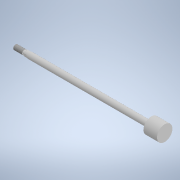
# Autodesk Inventor part: 32121200-s3
Saved by Autodesk Inventor 2024.3 (Build 283343000, 343)
## iProperties
Category: PARTsolutions
Company: METALWORK
Created: 2025-06-08
Part Number: 32121200-s3
Material: Generic
Catalog Web Link: www.cadenas.de
Description: ISO 15552 Type A rod-
Vendor: METALWORK
Document SubType Name: Modeling
Designer: psAdmin
Manufacturer: METALWORK
Mass: 53.2784 g
Surface Area: 148.649 cm^2
Volume: 53.2784 cm^3
Density: 1 g/cm^3
Appearance: PSOLRGB-175-175-175
PSOL_IDENT_0: {$CADENAS_DATA/23d-libs/metalwork/actuators/cyl_ser_iso_15552/series_3_conf/parts/iso_15552_a_rod.pr
PSOL_IDENT_1: j},191 {VTYP=3D},{NB=32121200-s3},{LINA=32121200-s3},{NN=ISO 15552 Type A rod},{DATE=01.09.2023 09:4
PSOL_IDENT_2: 1:06},{GEOMDATE=10.07.2023 09:16:00},{VERSION=},{LINEID=10},{WBVAR=TYPE,HUB,VER},{WBNUMERIC=HUB}  {N
PSOL_IDENT_3: B=32121200-s3},{LINA=32121200-s3},{KT=DUMMY},{DI=32},{TYPE=121},{TX= '121','Double-acting, cushioned'
PSOL_IDENT_4: , '122','Through-rod', '124','Double-acting, non-cuschioned', '125','Opposed', '126','Single-acting'
PSOL_IDENT_5: , '127','Tandem', '134','Rod lock version', '136','Version with piston rod lock','137','Piston rod l
PSOL_IDENT_6: ock + guide unit','154','Version suitable for bellow','156','Version with mounted bellow' },{HUB=200
PSOL_IDENT_7: },{HUBX=[1:2800]},{VER=},{VERX='','N/A'},{L=294.000},{LA=94.000},{LB=243.000},{L01=26.000},{L02=7.00
PSOL_IDENT_8: 0},{D=12.000},{D1=8.000},{D2=11.000},{PL=28.000},{PL1=28.000},{D2L=8.000},{WH=26.000},{WHX=26.000},{
PSOL_IDENT_9: C1=16.000},{F=22.000},{CH1=10.000},{CH1L=6.000},{RBL=58.000},{ND=10.000},{P=1.250},{L137=74.0},{L154=
PSOL_IDENT_10: 0},{WH154=0}
NB: 32121200-s3
NN: ISO 15552 Type A rod
NBSYN: $DI.$TYPE.$HUB.$VER.-s3
LINA: 32121200-s3
CATALOG: Metalwork
DI: 32
TYPE: Double-acting, cushioned
HUB: 200
VER: N/A
LB: 243
L01: 26
L02: 7
D: 12
D1: 8
D2: 11
PL1: 28
D2L: 8
WHX: 26
C1: 16
F: 22
CH1: 10
CH1L: 6
RBL: 58
ND: 10
P: 1.25
L137: 74
SUPPLIER: METALWORK
ARTICLENO: 32121200-s3
BOMINFO: 32121200-s3
CREATOR: CADENAS GmbH
Title: 32121200-s3
Author: Cadenas PARTsolutions
Autodesk Inventor part; units mm, degrees
sketch "Sketch_1" plane through (0, 0, 0) normal (0, 0, 1) x (1, 0, 0)
  line L0 (261, 0) -> (-48, 0)
  line L1 (-48, 0) -> (-48, 4.233)
  line L2 (-48, 4.233) -> (-47.233, 5)
  line L3 (-47.233, 5) -> (-29, 5)
  line L4 (-29, 5) -> (-29, 4)
  line L5 (-29, 4) -> (-26, 4)
  line L6 (-26, 4) -> (-26, 4.95)
  line L7 (-26, 4.95) -> (-25.45, 5.5)
  line L8 (-25.45, 5.5) -> (-18, 5.5)
  line L9 (-18, 5.5) -> (-18, 6)
  line L10 (-18, 6) -> (233, 6)
  line L11 (233, 6) -> (233, 16)
  line L12 (233, 16) -> (261, 16)
  line L13 (261, 16) -> (261, 0)
  line L14 (261, 0) -> (-48, 0)
  constraints: 30 end point
revolve "Revolution1" add sketch "Sketch_1" angle 360 about axis through (261, 0, 0) along (1, 0, 0)
thread "Thread1" size "M10x1.25" class "6g" standard "ISO Metric profile" full length
sketch "Sketch_3" plane through (-26, 0, 0) normal (1, 0, 0) x (0, 0, -1)
  line L0 (-10, -20) -> (10, -20)
  line L1 (10, -20) -> (10, 20)
  line L2 (10, 20) -> (-10, 20)
  line L3 (-10, 20) -> (-10, -20)
  line L4 (-5, -10) -> (5, -10)
  line L5 (5, -10) -> (5, 10)
  line L6 (5, 10) -> (-5, 10)
  line L7 (-5, 10) -> (-5, -10)
  constraints: 16 end point
extrude "Extrusion1" cut sketch "Sketch_3" along normal blind 6
ref_plane "accessories_l_XY" through (-38.5, 0, 0) normal (-1, 0, 0) x (0, 0, -1)
ref_plane "accessories_l_YZ" through (-38.5, 0, 0) normal (0, 0, -1) x (0, -1, 0)
ref_plane "accessories_l_ZX" through (-38.5, 0, 0) normal (0, -1, 0) x (-1, 0, 0)
ref_plane "rod_XY" through (0, 0, 0) normal (1, 0, 0) x (0, 0, -1)
ref_plane "rod_YZ" through (0, 0, 0) normal (0, 0, -1) x (0, 1, 0)
ref_plane "rod_ZX" through (0, 0, 0) normal (0, 1, 0) x (1, 0, 0)
body "Solid1"
